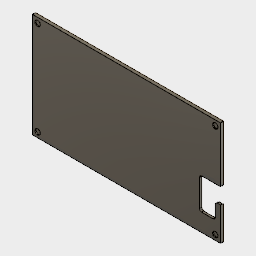
dock_backplate (Autodesk Fusion 360 design; units mm, degrees)
Autodesk Fusion 360 part; units mm, degrees
note: some values were not read from the file. Set by a fixed rule: which sketch regions a step uses.
sketch "Sketch1" plane through (0, 0, 0) normal (0, 0, 1) x (1, 0, 0)
  line L0 (0, 0) -> (170, 0)
  line L1 (170, 0) -> (170, 90)
  line L2 (170, 90) -> (0, 90)
  line L3 (0, 90) -> (0, 0)
  dimension "d1" = 170
  dimension "d2" = 90
  measures "d1" distance of L0.start L0.end
  measures "d2" distance of L0.start L2.end
extrude "Extrude1" add sketch "Sketch1" along normal blind 3
sketch "Sketch2" plane through (0, 0, 3) normal (0, 0, 1) x (1, 0, 0)
  line L0 (0, 90) -> (0, 0)
  line L1 (0, 0) -> (170, 0)
  line L2 (170, 0) -> (170, 90)
  line L3 (170, 90) -> (0, 90)
  line L4 (0, 0) -> (-5, 0)
  line L5 (-5, 0) -> (-5, -5)
  line L6 (-5, -5) -> (0, -5)
  line L7 (0, -5) -> (0, 0)
  line L8 (170, 90) -> (175, 90)
  line L9 (175, 90) -> (175, 95)
  line L10 (175, 95) -> (170, 95)
  line L11 (170, 95) -> (170, 90)
  line L12 (175, 95) -> (-5, 95)
  line L13 (-5, 95) -> (-5, -5)
  line L14 (-5, -5) -> (175, -5)
  line L15 (175, -5) -> (175, 95)
  dimension "d5" = 5
  dimension "d6" = 5
  dimension "d7" = 5
  dimension "d8" = 5
  measures "d5" distance of L0.end L4.end
  measures "d6" distance of L0.end L6.end
  measures "d7" distance of L2.end L10.end
  measures "d8" distance of L2.end L8.end
extrude "Extrude2" add sketch "Sketch2" against normal blind 3 contours L0 L3 L4 L11 L12 L13 | L4 L5 L6 L7 L13 L14 | L1 L2 L7 L8 L14 L15 | L8 L9 L10 L11 L12 L15
sketch "Sketch3" plane through (0, 0, 3) normal (0, 0, 1) x (1, 0, 0)
  line L0 (175, -5) -> (175, 95)
  line L1 (175, 95) -> (-5, 95)
  line L2 (-5, 95) -> (-5, -5)
  line L3 (-5, -5) -> (175, -5)
  line L4 (175, -5) -> (175, 27)
  line L5 (175, 27) -> (155, 27)
  line L6 (155, 27) -> (155, 42)
  line L7 (155, 42) -> (175, 42)
  line L8 (175, 42) -> (175, 27)
  line L9 (155, 27) -> (170, 27)
  line L10 (170, 27) -> (170, 12)
  line L11 (170, 12) -> (155, 12)
  line L12 (155, 12) -> (155, 27)
  dimension "d12" = 32
  dimension "d13" = 20
  dimension "d14" = 15
  dimension "d15" = 15
  dimension "d16" = 15
  measures "d12" distance of L0.start L4.end
  measures "d13" distance of L4.end L5.end
  measures "d14" distance of L4.end L7.end
  measures "d15" distance of L5.end L9.end
  measures "d16" distance of L5.end L11.end
extrude "Extrude3" cut sketch "Sketch3" against normal blind 5 contours L0 L5 L6 L7 L8 L9 | L5 L9 L10 L11 L12
fillet "Fillet1" radius 2 3 edges at (155, 12, 1.5) (170, 27, 1.5) (155, 42, 1.5)
fillet "Fillet2" radius 2 1 edges at (170, 12, 1.5)
fillet "Fillet3" radius 1 9 edges at (166, 42, 0) (155.5858, 41.4142, 0) (155, 27, 0) (155.5858, 12.5858, 0) (162.5, 12, 0) (169.4142, 12.5858, 0) (170, 19.5, 0) (170.5858, 26.4142, 0) (173.5, 27, 0)
sketch "Sketch4" plane through (0, 0, 0) normal (0, 0, -1) x (-1, 0, 0)
  line L0 (-172, 26) -> (-175, 26)
  line L1 (-175, 26) -> (-175, -5)
  line L2 (-175, -5) -> (5, -5)
  line L3 (5, -5) -> (5, 95)
  line L4 (5, 95) -> (-175, 95)
  line L5 (-175, 95) -> (-175, 43)
  line L6 (-175, 43) -> (-157, 43)
  arc A0 (-154, 40) -> (-157, 43) centre (-157, 40) ccw
  line L7 (-154, 40) -> (-154, 14)
  arc A1 (-157, 11) -> (-154, 14) centre (-157, 14) ccw
  line L8 (-157, 11) -> (-168, 11)
  arc A2 (-171, 14) -> (-168, 11) centre (-168, 14) ccw
  line L9 (-171, 14) -> (-171, 25)
  arc A3 (-171, 25) -> (-172, 26) centre (-172, 25) ccw
sketch "Sketch5" plane through (0, 0, 0) normal (0, 0, -1) x (-1, 0, 0)
  line L0 (-116, 50) -> (-116, 59.5)
  line L1 (-116, 59.5) -> (-113.5, 59.5)
  line L2 (-113.5, 59.5) -> (-109.2307, 53.1661)
  line L3 (-109.2307, 53.1661) -> (-109.2307, 59.5)
  line L4 (-109.2307, 59.5) -> (-106.5, 59.5)
  line L5 (-106.5, 59.5) -> (-106.5, 50.2404)
  line L6 (-106.5, 50.2404) -> (-109.2307, 50.2404)
  line L7 (-109.2307, 50.2404) -> (-113.5, 57)
  line L8 (-113.5, 57) -> (-113.5, 50.2404)
  line L9 (-113.5, 50.2404) -> (-113.5, 50)
  line L10 (-113.5, 50) -> (-116, 50)
  line L11 (-102.8507, 59.4444) -> (-105.7917, 59.4444)
  line L12 (-105.7917, 59.4444) -> (-105.7917, 57.5559)
  line L13 (-105.7917, 57.5559) -> (-102.8507, 57.5559)
  line L14 (-102.8507, 57.5559) -> (-102.8507, 59.4444)
  line L15 (-105.7917, 56.395) -> (-102.8507, 56.395)
  line L16 (-102.8507, 56.395) -> (-102.8507, 50.1491)
  line L17 (-102.8507, 50.1491) -> (-105.7917, 50.1491)
  line L18 (-105.7917, 50.1491) -> (-105.7917, 56.395)
  line L19 (-101.8554, 50.1491) -> (-99, 50.1491)
  line L20 (-99, 50.1491) -> (-99, 56.5)
  line L21 (-99, 56.5) -> (-101.8554, 56.5)
  line L22 (-101.8554, 56.5) -> (-101.8554, 50.1491)
  line L23 (-86.3188, 57.5559) -> (-83.3127, 57.5559)
  line L24 (-83.3127, 57.5559) -> (-83.3127, 59.4542)
  line L25 (-83.3127, 59.4542) -> (-86.3188, 59.4542)
  line L26 (-86.3188, 59.4542) -> (-86.3188, 57.5559)
  line L27 (-86.3188, 56.5) -> (-83.3127, 56.5)
  line L28 (-83.3127, 56.5) -> (-83.3127, 50.1753)
  line L29 (-83.3127, 50.1753) -> (-86.3188, 50.1753)
  line L30 (-86.3188, 50.1753) -> (-86.3188, 56.5)
  line L31 (-82.3817, 50.1753) -> (-80.097, 50.1753)
  line L32 (-80.097, 50.1753) -> (-80.097, 56.5)
  line L33 (-80.097, 56.5) -> (-82.3817, 56.5)
  line L34 (-82.3817, 56.5) -> (-82.3817, 50.1753)
  line L35 (-62.3862, 50.1753) -> (-65.0316, 50.1753)
  line L36 (-65.0316, 50.1753) -> (-65.0316, 59.7132)
  line L37 (-65.0316, 59.7132) -> (-62.3862, 59.7132)
  line L38 (-62.3862, 59.7132) -> (-62.3862, 50.1753)
  line L39 (-91.2154, 50.1753) -> (-88.7237, 50.1753)
  line L40 (-88.7237, 50.1753) -> (-88.7237, 58.3516)
  line L41 (-88.7237, 58.3516) -> (-91.2154, 58.3516)
  line L42 (-91.2154, 58.3516) -> (-91.2154, 50.1753)
  line L43 (-92.9, 57) -> (-87, 57)
  line L44 (-87, 57) -> (-87, 55.9)
  line L45 (-87, 55.9) -> (-92.9, 55.9)
  line L46 (-92.9, 55.9) -> (-92.9, 57)
  line L47 (-93.8, 50.1) -> (-96.5047, 50.1)
  line L48 (-96.5047, 50.1) -> (-96.5047, 54.9443)
  line L49 (-96.5047, 54.9443) -> (-93.8, 54.9443)
  line L50 (-93.8, 54.9443) -> (-93.8, 50.1)
  line L51 (-75.5551, 50.1) -> (-77.9127, 50.1)
  line L52 (-77.9127, 50.1) -> (-77.9127, 54.9443)
  line L53 (-77.9127, 54.9443) -> (-75.5551, 54.9443)
  line L54 (-75.5551, 54.9443) -> (-75.5551, 50.1)
  line L55 (-70.7736, 50.1) -> (-73, 50.1)
  line L56 (-73, 50.1) -> (-73, 54.5)
  line L57 (-73, 54.5) -> (-70.7736, 54.5)
  line L58 (-70.7736, 54.5) -> (-70.7736, 50.1)
  line L59 (-77.9127, 54.9443) -> (-78.1822, 55.3355)
  line L60 (-78.1822, 55.3355) -> (-78.7771, 55.6219)
  line L61 (-78.7771, 55.6219) -> (-79.5, 55.6219)
  line L62 (-79.5, 55.6219) -> (-80.097, 54.9443)
  line L63 (-80.097, 55.7651) -> (-79.5, 56.24)
  line L64 (-79.5, 56.24) -> (-78.7771, 56.606)
  line L65 (-78.7771, 56.606) -> (-78.1, 56.8)
  line L66 (-78.1, 56.8) -> (-77.3, 56.8)
  line L67 (-77.3, 56.8) -> (-76.522, 56.703)
  line L68 (-76.522, 56.703) -> (-76.1, 56.4)
  line L69 (-76.1, 56.4) -> (-75.8, 55.9)
  line L70 (-75.8, 55.9) -> (-75.6113, 55.5854)
  line L71 (-75.6113, 55.5854) -> (-74.9, 56.2)
  line L72 (-74.9, 56.2) -> (-74.456, 56.5836)
  line L73 (-74.456, 56.5836) -> (-73.8, 56.8)
  line L74 (-73.8, 56.8) -> (-73.1367, 56.99)
  line L75 (-73.1367, 56.99) -> (-72.4898, 56.9094)
  line L76 (-72.4898, 56.9094) -> (-71.7871, 56.7515)
  line L77 (-71.7871, 56.7515) -> (-71.3, 56.3)
  line L78 (-71.3, 56.3) -> (-70.9, 55.7)
  line L79 (-70.9, 55.7) -> (-70.7407, 55.1439)
  line L80 (-70.7407, 55.1439) -> (-70.7736, 54.5)
  line L81 (-73, 54.5) -> (-73.1257, 54.9388)
  line L82 (-73.1257, 54.9388) -> (-73.5, 55.3)
  line L83 (-73.5, 55.3) -> (-74.1, 55.4)
  line L84 (-74.1, 55.4) -> (-74.7056, 55.35)
  line L85 (-74.7056, 55.35) -> (-75.3, 55)
  line L86 (-75.3, 55) -> (-75.5551, 54.9443)
  line L87 (-96.5047, 54.9443) -> (-96.7728, 55.375)
  line L88 (-96.7728, 55.375) -> (-97.3, 55.5)
  line L89 (-97.3, 55.5) -> (-97.8554, 55.6317)
  line L90 (-97.8554, 55.6317) -> (-98.5, 55.5)
  line L91 (-98.5, 55.5) -> (-99, 54.9779)
  line L92 (-99, 55.9042) -> (-97.8, 56.6)
  line L93 (-97.8, 56.6) -> (-96.6839, 56.828)
  line L94 (-96.6839, 56.828) -> (-95.4, 56.828)
  line L95 (-95.4, 56.828) -> (-94.5, 56.3)
  line L96 (-94.5, 56.3) -> (-93.9, 55.5)
  line L97 (-93.9, 55.5) -> (-93.8, 54.9443)
  line L98 (-65.0316, 50.5) -> (-65.5721, 50.1753)
  line L99 (-65.5721, 50.1753) -> (-67.7799, 50.1753)
  line L100 (-67.7799, 50.1753) -> (-68.9927, 50.7177)
  line L101 (-68.9927, 50.7177) -> (-70, 52)
  line L102 (-70, 52) -> (-70.1899, 53.4853)
  line L103 (-70.1899, 53.4853) -> (-69.8012, 54.9443)
  line L104 (-69.8012, 54.9443) -> (-68.8372, 56.1751)
  line L105 (-68.8372, 56.1751) -> (-67.5001, 56.766)
  line L106 (-67.5001, 56.766) -> (-65.8519, 56.766)
  line L107 (-65.8519, 56.766) -> (-65.0316, 56.3991)
  line L108 (-61.7902, 53.6059) -> (-61.4948, 54.9443)
  line L109 (-61.4948, 54.9443) -> (-60.6707, 56.0004)
  line L110 (-60.6707, 56.0004) -> (-59.1632, 56.6665)
  line L111 (-59.1632, 56.6665) -> (-57.2811, 56.766)
  line L112 (-57.2811, 56.766) -> (-55.6797, 56.3334)
  line L113 (-55.6797, 56.3334) -> (-54.5757, 55.2851)
  line L114 (-54.5757, 55.2851) -> (-54.187, 53.9635)
  line L115 (-54.187, 53.9635) -> (-54.187, 52.7352)
  line L116 (-54.187, 52.7352) -> (-54.5757, 51.6002)
  line L117 (-54.5757, 51.6002) -> (-56, 50.5)
  line L118 (-56, 50.5) -> (-57.7942, 50.1697)
  line L119 (-57.7942, 50.1697) -> (-59.5, 50.5)
  line L120 (-59.5, 50.5) -> (-61, 51.5)
  line L121 (-61, 51.5) -> (-61.6502, 52.5797)
  line L122 (-61.6502, 52.5797) -> (-61.7902, 53.6059)
  arc A0 (-65.0316, 55.206) -> (-67.179, 55.1361) centre (-66.0986, 54.9647) ccw
  arc A1 (-67.179, 52.0056) -> (-65.0316, 52.0755) centre (-66.1064, 52.0755) ccw
  arc A2 (-56.8264, 54.9443) -> (-59.0904, 54.9443) centre (-57.9584, 54.9347) ccw
  arc A3 (-59.0904, 52.0082) -> (-56.8543, 52.0082) centre (-57.9723, 52.1253) ccw
  line L123 (-59.0904, 54.9443) -> (-59.0904, 52.0082)
  line L124 (-56.8264, 54.9443) -> (-56.8543, 52.0082)
  line L125 (-67.179, 55.1361) -> (-67.179, 52.0056)
  circle A4 centre (-51.9221, 58.0784) radius 1.4242
  line L126 (-116, 62.479) -> (-54, 62.479)
  line L127 (-54, 62.479) -> (-54, 65)
  line L128 (-54, 65) -> (-116, 65)
  line L129 (-116, 65) -> (-116, 62.479)
  line L130 (-116, 65) -> (-54, 65)
  line L131 (-54, 45) -> (-116, 45)
  line L132 (-54, 45) -> (-116, 45)
  line L133 (-116, 45) -> (-116, 47.521)
  line L134 (-116, 47.521) -> (-54, 47.521)
  line L135 (-54, 47.521) -> (-54, 45)
  arc A5 (-116, 62.479) -> (-116, 47.521) centre (-116, 55) ccw
  arc A6 (-116, 65) -> (-116, 45) centre (-116, 55) ccw
  arc A7 (-54, 47.521) -> (-54, 62.479) centre (-54, 55) ccw
  arc A8 (-54, 45) -> (-54, 65) centre (-54, 55) ccw
  dimension "d22" = 2.521
  measures "d22" distance of L131.start L134.end
extrude "Extrude4" cut sketch "Sketch5" against normal blind 1 contours L0 L1 L2 L3 L4 L5 L6 L7 L8 L9 L10 | L11 L12 L13 L14 | L15 L16 L17 L18 | L19 L20 L21 L22 | L20 L49 L87 L88 L89 L90 L91 L92 L93 L94 L95 L96 L97 | L47 L48 L49 L50 | L23 L24 L25 L26 | L27 L28 L29 L30 | L31 L32 L33 L34 | L32 L53 L57 L59 L60 L61 L62 L63 L64 L65 L66 L67 L68 L69 L70 L71 L72 L73 L74 L75 L76 L77 L78 L79 L80 L81 L82 L83 L84 L85 L86 | L51 L52 L53 L54 | L55 L56 L57 L58 | L35 L36 L37 L38 | L36 L98 L99 L100 L101 L102 L103 L104 L105 L106 L107 A0 A1 L125 | L39 L40 L42 L45 | L42 L43 L45 L46 | L40 L42 L43 L45 | L40 L43 L44 L45 | L40 L41 L42 L43 | L108 L109 L110 L111 L112 L113 L114 L115 L116 L117 L118 L119 L120 L121 L122 | A4 | L126 L127 L128 L129 L130 | L129 L133 A5 A6 | L127 L135 A7 A8 | L131 L132 L133 L134 L135
sketch "Sketch6" plane through (0, 0, 3) normal (0, 0, 1) x (1, 0, 0)
  arc A0 (172, 27) -> (170, 25) centre (172, 25) ccw
  line L0 (170, 25) -> (170, 14)
  arc A1 (168, 12) -> (170, 14) centre (168, 14) ccw
  line L1 (168, 12) -> (157, 12)
  arc A2 (155, 14) -> (157, 12) centre (157, 14) ccw
  line L2 (155, 14) -> (155, 40)
  arc A3 (157, 42) -> (155, 40) centre (157, 40) ccw
  line L3 (157, 42) -> (175, 42)
  line L4 (175, 42) -> (175, 95)
  line L5 (175, 95) -> (-5, 95)
  line L6 (-5, 95) -> (-5, -5)
  line L7 (-5, -5) -> (175, -5)
  line L8 (175, -5) -> (175, 27)
  line L9 (175, 27) -> (172, 27)
  line L10 (-5, 95) -> (0, 95)
  line L11 (0, 95) -> (0, 90)
  line L12 (0, 90) -> (-5, 90)
  line L13 (-5, 90) -> (-5, 95)
  line L14 (175, 95) -> (170, 95)
  line L15 (170, 95) -> (170, 90)
  line L16 (170, 90) -> (175, 90)
  line L17 (175, 90) -> (175, 95)
  line L18 (175, -5) -> (170, -5)
  line L19 (170, -5) -> (170, 0)
  line L20 (170, 0) -> (175, 0)
  line L21 (175, 0) -> (175, -5)
  line L22 (-5, -5) -> (0, -5)
  line L23 (0, -5) -> (0, 0)
  line L24 (0, 0) -> (-5, 0)
  line L25 (-5, 0) -> (-5, -5)
  circle A4 centre (0, 0) radius 2.6
  circle A5 centre (0, 90) radius 2.6
  circle A6 centre (170, 90) radius 2.6
  circle A7 centre (170, 0) radius 2.6
  dimension "d25" = 5
  dimension "d26" = 5.2
  dimension "d27" = 5.2
  dimension "d28" = 5.2
  dimension "d29" = 5.2
  measures "d25" distance of L5.end L12.end
  measures "d26" diameter of A4
  measures "d27" diameter of A5
  measures "d28" diameter of A6
  measures "d29" diameter of A7
extrude "Extrude5" cut sketch "Sketch6" against normal blind 1 contours L19 L20 A7 | L19 L20 A7 | L23 L24 A4 | L23 L24 A4 | L11 L12 A5 | L11 L12 A5 | L15 L16 A6 | L15 L16 A6
